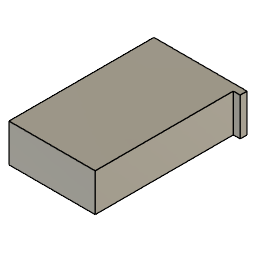
NovaHub (Autodesk Fusion 360 archive; units mm, degrees)
design "Meshnology Battery"
Autodesk Fusion 360 part; units mm, degrees
sketch "Sketch1" plane through (0, 0, 0) normal (0, 0, 1) x (1, 0, 0)
  line L0 (12.5, 21) -> (-12.5, 21)
  line L1 (-12.5, 21) -> (-12.5, -21)
  line L2 (-12.5, -21) -> (12.5, -21)
  line L3 (12.5, -21) -> (12.5, 21)
  line L4 (12.5, 21) -> (-12.5, -21) construction
  line L5 (-12.5, 21) -> (12.5, -21) construction
  line L6 (12.5, 21) -> (14.5, 21)
  line L7 (14.5, 21) -> (14.5, 19)
  line L8 (14.5, 19) -> (12.5, 19)
  line L9 (12.5, 19) -> (12.5, 21)
  dimension "d1" = 25
  dimension "d2" = 42
  dimension "d3" = 2
  dimension "d4" = 2
  constraint horizontal L0
  constraint perpendicular L0 L1
  constraint parallel L0 L2
  constraint parallel L1 L3
  constraint coincident L4 origin
  constraint coincident L5 origin
  constraint horizontal L6
  constraint vertical L7
  constraint horizontal L8
  constraint vertical L9
  measures "d1" distance of L1.end L2.end
  measures "d2" distance of L0.end L1.end
  measures "d3" distance of L0.start L6.end
  measures "d4" distance of L0.start L8.end
extrude "Extrude1" add sketch "Sketch1" along normal blind 11

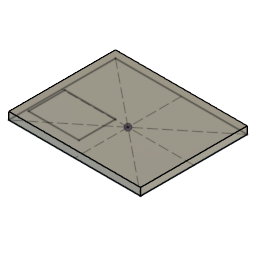
design "433 Transmitter"
Autodesk Fusion 360 part; units mm, degrees
sketch "Sketch1" plane through (0, 0, 0) normal (0, 0, 1) x (1, 0, 0)
  line L0 (15, 12.15) -> (-15, 12.15)
  line L1 (-15, 12.15) -> (-15, -12.15)
  line L2 (-15, -12.15) -> (15, -12.15)
  line L3 (15, -12.15) -> (15, 12.15)
  line L4 (15, 12.15) -> (-15, -12.15) construction
  line L5 (-15, 12.15) -> (15, -12.15) construction
  line L6 (-14.5, 0.15) -> (-3, 0.15)
  line L7 (-3, 0.15) -> (-3, -8.15)
  line L8 (-3, -8.15) -> (-14.5, -8.15)
  line L9 (-14.5, -8.15) -> (-14.5, 0.15)
  line L10 (15, 0) -> (-15, 0) construction
  line L11 (0, 12.15) -> (0, -12.15) construction
  dimension "d1" = 30
  dimension "d2" = 24.3
  dimension "d5" = 12
  dimension "d6" = 4
  dimension "d7" = 18
  dimension "d8" = 0.5
  constraint horizontal L0
  constraint perpendicular L0 L1
  constraint parallel L0 L2
  constraint parallel L1 L3
  constraint coincident L4 origin
  constraint coincident L5 origin
  constraint horizontal L6
  constraint vertical L7
  constraint horizontal L8
  constraint vertical L9
  constraint midpoint L3 L10.start
  constraint midpoint L1 L10.end
  constraint midpoint L0 L11.start
  constraint midpoint L2 L11.end
  measures "d1" distance of L1.end L2.end
  measures "d2" distance of L0.end L1.end
  measures "d5" distance of L0 L6
  measures "d6" distance of L2 L8
  measures "d7" distance of L3 L7
  measures "d8" distance of L1 L9
extrude "Extrude1" add sketch "Sketch1" along normal blind 1.7 contours L0 L1 L2 L3 | L6 L7 L8 L9
extrude "Extrude2" add sketch "Sketch1" against normal blind 2 contours L6 L7 L8 L9

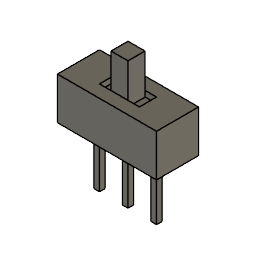
design "Switch"
Autodesk Fusion 360 part; units mm, degrees
sketch "Sketch1" plane through (0, 0, 0) normal (0, 0, 1) x (1, 0, 0)
  line L0 (4.35, -1.85) -> (-4.35, -1.85)
  line L1 (-4.35, -1.85) -> (-4.35, 1.85)
  line L2 (-4.35, 1.85) -> (4.35, 1.85)
  line L3 (4.35, 1.85) -> (4.35, -1.85)
  line L4 (4.35, -1.85) -> (-4.35, 1.85) construction
  line L5 (-4.35, -1.85) -> (4.35, 1.85) construction
  line L6 (0.75, 0.75) -> (-0.75, 0.75)
  line L7 (-0.75, 0.75) -> (-0.75, -0.75)
  line L8 (-0.75, -0.75) -> (0.75, -0.75)
  line L9 (0.75, -0.75) -> (0.75, 0.75)
  line L10 (0.75, 0.75) -> (-0.75, -0.75) construction
  line L11 (-0.75, 0.75) -> (0.75, -0.75) construction
  line L12 (-1.75, 0.75) -> (1.75, 0.75)
  line L13 (1.75, 0.75) -> (1.75, -0.75)
  line L14 (1.75, -0.75) -> (-1.75, -0.75)
  line L15 (-1.75, -0.75) -> (-1.75, 0.75)
  line L16 (-2.25, 0.25) -> (-2.75, 0.25)
  line L17 (-2.75, 0.25) -> (-2.75, -0.25)
  line L18 (-2.75, -0.25) -> (-2.25, -0.25)
  line L19 (-2.25, -0.25) -> (-2.25, 0.25)
  line L20 (-2.25, 0.25) -> (-2.75, -0.25) construction
  line L21 (-2.75, 0.25) -> (-2.25, -0.25) construction
  line L22 (0.25, -0.25) -> (0.25, 0.25)
  line L23 (0.25, 0.25) -> (-0.25, -0.25) construction
  line L24 (-0.25, 0.25) -> (0.25, -0.25) construction
  line L25 (-0.25, 0.25) -> (-0.25, -0.25)
  line L26 (0.25, 0.25) -> (-0.25, 0.25)
  line L27 (-0.25, -0.25) -> (0.25, -0.25)
  line L28 (2.75, -0.25) -> (2.75, 0.25)
  line L29 (2.75, 0.25) -> (2.25, -0.25) construction
  line L30 (2.25, 0.25) -> (2.75, -0.25) construction
  line L31 (2.25, 0.25) -> (2.25, -0.25)
  line L32 (2.75, 0.25) -> (2.25, 0.25)
  line L33 (2.25, -0.25) -> (2.75, -0.25)
  point P0 (-2.5, 0)
  point P1 (2.5, 0)
  dimension "d1" = 8.7
  dimension "d2" = 3.7
  dimension "d3" = 1.5
  dimension "d4" = 1.5
  dimension "d5" = 3.5
  dimension "d6" = 0.5
  dimension "d7" = 0.5
  dimension "d8" = 0.5
  dimension "d9" = 0.5
  dimension "d10" = 0.5
  dimension "d11" = 0.5
  dimension "d12" = 2.5
  dimension "d13" = 2.5
  constraint horizontal L0
  constraint perpendicular L0 L1
  constraint parallel L0 L2
  constraint parallel L1 L3
  constraint coincident L4 origin
  constraint coincident L5 origin
  constraint horizontal L6
  constraint perpendicular L6 L7
  constraint parallel L6 L8
  constraint parallel L7 L9
  constraint coincident L10 origin
  constraint coincident L11 origin
  constraint horizontal L12
  constraint vertical L13
  constraint horizontal L14
  constraint vertical L15
  constraint midpoint L6 L12
  constraint midpoint L8 L14
  constraint horizontal L16
  constraint perpendicular L16 L17
  constraint parallel L16 L18
  constraint parallel L17 L19
  constraint coincident L20 P0
  constraint coincident L21 P0
  constraint horizontal L26
  constraint perpendicular L25 L26
  constraint parallel L26 L27
  constraint parallel L22 L25
  constraint coincident origin L23
  constraint coincident origin L24
  constraint horizontal L32
  constraint perpendicular L31 L32
  constraint parallel L32 L33
  constraint parallel L28 L31
  constraint coincident P1 L29
  constraint coincident P1 L30
  constraint horizontal origin P1
  constraint horizontal origin P0
  measures "d1" distance of L1.end L2.end
  measures "d2" distance of L0.end L1.end
  measures "d3" distance of L7.end L8.end
  measures "d4" distance of L6.end L7.end
  measures "d5" distance of L12.start L12.end
  measures "d6" distance of L17.end L18.end
  measures "d7" distance of L16.end L17.end
  measures "d8" distance of L23.end L22.start
  measures "d9" distance of L24.start L23.end
  measures "d10" distance of L29.end L28.start
  measures "d11" distance of L30.start L29.end
  measures "d12" distance of origin P1
  measures "d13" distance of P0 origin
extrude "Extrude1" add sketch "Sketch1" along normal blind 3.7 contours L0 L1 L2 L3 | L6 L7 L8 L9 L12 L14 | L9 L12 L13 L14 | L7 L12 L14 L15 | L16 L17 L18 L19 | L22 L25 L26 L27 | L28 L31 L32 L33
extrude "Extrude2" cut sketch "Sketch1" against normal blind 0.5 from surface at 3.7 contours L6 L7 L8 L9 L12 L14 | L9 L12 L13 L14 | L7 L12 L14 L15 | L22 L25 L26 L27
extrude "Extrude3" add sketch "Sketch1" along normal blind 3 and the other way up to surface (0.5 mm away) from surface at 3.7 contours L6 L7 L8 L9 L12 L14 | L22 L25 L26 L27
extrude "Extrude4" add sketch "Sketch1" against normal blind 5 contours L16 L17 L18 L19 | L22 L25 L26 L27 | L28 L31 L32 L33
